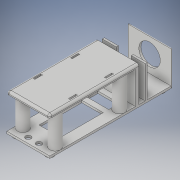
# Autodesk Inventor part: TestingPlatform
Saved by Autodesk Inventor 2017 (Build 210142000, 142)
## iProperties
Created: 2018-05-20
Part Number: TestingPlatform
Material: Generic
Document SubType Name: Modeling
Designer: Arthur
Density: 1 g/cm^3
Appearance: Default
Author: Arthur
Autodesk Inventor part; units mm, degrees
ref_plane "YZ Plane" through (0, 0, 0) normal (1, 0, 0) x (0, 1, 0)
ref_plane "XZ Plane" through (0, 0, 0) normal (0, 1, 0) x (-1, 0, 0)
ref_plane "XY Plane" through (0, 0, 0) normal (0, 0, 1) x (1, 0, 0)
sketch "Sketch1" plane through (0, 0, 0) normal (0, 1, 0) x (-1, 0, 0)
  line L0 (-20, 57.5) -> (20, 57.5)
  line L1 (20, 57.5) -> (20, -57.5)
  line L2 (20, -57.5) -> (-20, -57.5)
  line L3 (-20, -57.5) -> (-20, 57.5)
  line L4 (-20, 57.5) -> (20, -57.5) construction
  line L5 (20, 57.5) -> (-20, -57.5) construction
  point P0 (0, 0)
  dimension "d0" = 40
  dimension "d1" = 115
  constraints: 12 end point, 2 midpoint, 2 parallel, 1 horizontal, 1 perpendicular
  measures "d0" distance of L1.end L2.end
  measures "d1" distance of L0.end L1.end
extrude "Extrusion1" add sketch "Sketch1" along normal blind 2
sketch "Sketch3" plane through (0, 2, 0) normal (0, 1, 0) x (1, 0, 0)
  line L0 (-20, 57.5) -> (-20, -57.5) projected
  line L1 (-20, -57.5) -> (-20, -47.5)
  line L2 (-20, 22.4101) -> (-20, 12.4101)
  line L3 (-20, -47.5) -> (-15, -47.5)
  line L4 (-20, 12.4101) -> (-15, 12.4101)
  line L5 (20, -47.5) -> (15, -47.5)
  circle A0 centre (15, -47.5) radius 5
  circle A1 centre (15, 12.4101) radius 5
  line L6 (20, -57.5) -> (20, 57.5) projected
  circle A2 centre (-15, 12.4101) radius 5
  circle A3 centre (-15, -47.5) radius 5
  line L7 (-20, 22.4101) -> (20, 22.4101)
  line L8 (20, 22.4101) -> (20, 25.4101)
  line L9 (20, 25.4101) -> (-20, 25.4101)
  line L10 (-20, 25.4101) -> (-20, 22.4101)
  line L11 (-20, 25.4101) -> (-20, 31.4101)
  line L12 (-20, 31.4101) -> (-7, 31.4101)
  line L13 (-7, 31.4101) -> (-7, 33.4101)
  line L14 (-7, 33.4101) -> (-20, 33.4101)
  line L15 (-20, 33.4101) -> (-20, 31.4101)
  line L16 (20, 31.4101) -> (7, 31.4101)
  line L17 (7, 31.4101) -> (7, 33.4101)
  line L18 (7, 33.4101) -> (20, 33.4101)
  line L19 (20, 33.4101) -> (20, 31.4101)
  line L20 (20, 57.5) -> (-20, 57.5) projected
  line L21 (20, 57.5) -> (-20, 57.5)
  line L22 (-20, 57.5) -> (-20, 55.5)
  line L23 (-20, 55.5) -> (20, 55.5)
  line L24 (20, 55.5) -> (20, 57.5)
  point P0 (0, 0)
  dimension "d17" = 10
  dimension "d18" = 10
  dimension "d19" = 5
  dimension "d21" = 5
  dimension "d22" = 5
  dimension "d23" = 40
  dimension "d24" = 3
  dimension "d25" = 6
  dimension "d26" = 13
  dimension "d27" = 2
  dimension "d28" = 13
  dimension "d29" = 2
  dimension "d30" = 40
  dimension "d31" = 2
  constraints: 44 end point, 8 parallel, 7 horizontal, 5 point on line, 4 perpendicular, 3 coincident, 3 horizontal alignment, 1 centre point, 1 tangent, 6 other
  measures "d17" distance of L0.end L1.end
  measures "d18" distance of L2.start L2.end
  measures "d19" distance of L1.end L3.end
  measures "d21" distance of L2.end L4.end
  measures "d22" distance of L5.start L5.end
  measures "d23" distance of L9.end L8.end
  measures "d24" distance of L8.end L7.end
  measures "d25" distance of L9.end L11.end
  measures "d26" distance of L14.end L13.end
  measures "d27" distance of L13.end L12.end
  measures "d28" distance of L17.end L18.end
  measures "d29" distance of L16.end L17.end
  measures "d30" distance of L23.end L22.end
  measures "d31" distance of L22.end L21.end
extrude "Extrusion2" add sketch "Sketch3" along normal blind 30 contours L20 L6 L23 L0 | L14 L13 L12 L0 | L6 L16 L17 L18 | L9 L6 L7 L0 | A0 | A1 | A2 | A3
sketch "Sketch5" plane through (-15, 32, -12.4101) normal (0, 1, 0) x (1, 0, 0)
  line L0 (35, 13) -> (-5, 13) projected
  line L1 (35, 45.0899) -> (35, -69.9101) projected
  line L2 (-5, 13) -> (35, 13)
  line L3 (35, 13) -> (35, -69.9101)
  line L4 (35, -69.9101) -> (-5, -69.9101)
  line L5 (-5, -69.9101) -> (-5, 13)
  point P0 (15, -12.4101)
  constraints: 8 end point, 2 parallel, 1 horizontal, 1 perpendicular
extrude "Extrusion3" add sketch "Sketch5" along normal blind 3
sketch "Sketch6" plane through (20, 0, -57.5) normal (0, 0, -1) x (-1, 0, 0)
  line L0 (40, 35) -> (0, 35) projected
  circle A0 centre (20, 17.5) radius 10
  point P0 (20, 0)
  dimension "d37" = 20
  constraints: 1 centre point
  measures "d37" diameter of A0
extrude "Extrusion4" cut sketch "Sketch6" against normal blind 2
sketch "Sketch7" plane through (0, 2, 0) normal (0, 1, 0) x (1, 0, 0)
  line L0 (20, -47.5) -> (20, 12.4101) projected
  circle A0 centre (-15, -47.5) radius 5 projected
  line L1 (10, 2.4101) -> (-10, 2.4101)
  line L2 (-10, 2.4101) -> (-10, -37.5)
  line L3 (-10, -37.5) -> (10, -37.5)
  line L4 (10, -37.5) -> (10, 2.4101)
  point P0 (0, 0)
  point P1 (-20, -47.5)
  constraints: 8 end point, 2 parallel, 1 horizontal, 1 horizontal alignment, 1 perpendicular
extrude "Extrusion5" cut sketch "Sketch7" against normal through all contours L4 L3 L2 L1
fillet "Fillet1" radius 2 1 edges at (-20, 35, 16.045)
fillet "Fillet2" radius 2 1 edges at (20, 35, 16.045)
fillet "Fillet3" radius 2 3 edges at (0, 32, -57.5) (-20, 16, -57.5) (20, 16, -57.5)
fillet "Fillet4" radius 2 5 edges at (0, 35, 57.5) (19.4142, 34.4142, 57.5) (20, 32.5, 57.5) (-19.4142, 34.4142, 57.5) (-20, 32.5, 57.5)
sketch "Sketch8" plane through (0, 2, 0) normal (0, 1, 0) x (1, 0, 0)
  circle A0 centre (-15, -47.5) radius 5 projected
  circle A1 centre (-5, -52.5) radius 2.5
  circle A2 centre (15, -47.5) radius 5 projected
  circle A3 centre (5, -52.5) radius 2.5
  point P0 (0, 0)
  point P1 (-20, -47.5)
  point P2 (20, -47.5)
  dimension "d52" = 5
  dimension "d55" = 5
  constraints: 2 centre point, 2 horizontal alignment
  measures "d52" diameter of A1
  measures "d55" diameter of A3
extrude "Extrusion6" cut sketch "Sketch8" against normal through all contours A1 | A3
sketch "Sketch9" plane through (-15, 35, -12.4101) normal (0, 1, 0) x (1, 0, 0)
  line L0 (-3, -67.9101) -> (-3, 13) projected
  line L1 (-1, -7) -> (-1.5, -7)
  line L2 (-1.5, -7) -> (0, -7)
  line L3 (0, -7) -> (0, -14)
  line L4 (0, -14) -> (-1.5, -14)
  line L5 (-1.5, -14) -> (-1.5, -7)
  line L6 (31, -7) -> (31.5, -7)
  line L7 (31.5, -7) -> (30, -7)
  line L8 (30, -7) -> (30, -14)
  line L9 (30, -14) -> (31.5, -14)
  line L10 (31.5, -14) -> (31.5, -7)
  line L11 (-3, -67.9101) -> (-1.5, -67.9101)
  line L12 (33, -67.9101) -> (-3, -67.9101) projected
  line L13 (-1.5, -47.9101) -> (-2.25, -47.9101)
  line L14 (-2.25, -47.9101) -> (-0.75, -47.9101)
  line L15 (-0.75, -47.9101) -> (-0.75, -40.9101)
  line L16 (-0.75, -40.9101) -> (-2.25, -40.9101)
  line L17 (-2.25, -40.9101) -> (-2.25, -47.9101)
  line L18 (30.75, -47.9101) -> (31.875, -47.9101)
  line L19 (31.875, -47.9101) -> (30.375, -47.9101)
  line L20 (30.375, -47.9101) -> (30.375, -40.9101)
  line L21 (30.375, -40.9101) -> (31.875, -40.9101)
  line L22 (31.875, -40.9101) -> (31.875, -47.9101)
  point P0 (15, -12.4101)
  dimension "d61" = 1.5
  dimension "d62" = 7
  dimension "d65" = 1.5
  dimension "d66" = 7
  dimension "d68" = 1.5
  dimension "d69" = 7
  dimension "d71" = 1.5
  dimension "d72" = 7
  constraints: 42 end point, 8 parallel, 6 horizontal, 4 perpendicular, 1 point on line
  measures "d61" distance of L3.end L4.end
  measures "d62" distance of L2.end L3.end
  measures "d65" distance of L9.end L8.end
  measures "d66" distance of L8.end L7.end
  measures "d68" distance of L16.end L15.end
  measures "d69" distance of L15.end L14.end
  measures "d71" distance of L20.end L21.end
  measures "d72" distance of L19.end L20.end
extrude "Extrusion7" cut sketch "Sketch9" against normal blind 3
sketch "Sketch11" plane through (0, 2, 0) normal (0, 1, 0) x (1, 0, 0)
  line L0 (-10, -37.5) -> (-10, 2.4101) projected
  line L1 (10, 2.4101) -> (10, -37.5) projected
  line L2 (10, 7.4101) -> (-10, 7.4101)
  line L3 (-10, 7.4101) -> (-10, 17.4101)
  line L4 (-10, 17.4101) -> (10, 17.4101)
  line L5 (10, 17.4101) -> (10, 7.4101)
  point P0 (0, 0)
  dimension "d76" = 5
  dimension "d77" = 20
  dimension "d78" = 10
  constraints: 8 end point, 2 parallel, 1 horizontal, 1 perpendicular
  measures "d76" distance of L1.start L2.start
  measures "d77" distance of L3.end L4.end
  measures "d78" distance of L2.end L3.end
extrude "Extrusion8" cut sketch "Sketch11" against normal through all
sketch "Sketch12" plane through (0, 0, 0) normal (0, -1, 0) x (1, 0, 0)
  line L0 (20, -55.5) -> (-20, -55.5) projected
  line L1 (-20, -55.5) -> (-15, -55.5)
  line L2 (20, -55.5) -> (20, 57.5) projected
  line L3 (20, 57.5) -> (-20, 57.5) projected
  circle A0 centre (-15, 47.5) radius 5 projected
  circle A1 centre (15, 47.5) radius 5 projected
  circle A2 centre (-15, -50.5) radius 3.5
  circle A3 centre (15, -50.5) radius 3.5
  circle A4 centre (-15, 52.5) radius 3.5
  circle A5 centre (15, 52.5) radius 3.5
  point P0 (0, 0)
  point P1 (-20, 47.5)
  point P2 (20, 47.5)
  dimension "d88" = 7
  dimension "d89" = 7
  dimension "d90" = 7
  dimension "d91" = 7
  constraints: 4 centre point, 2 end point, 2 horizontal alignment, 1 point on line
  measures "d88" diameter of A2
  measures "d89" diameter of A3
  measures "d90" diameter of A4
  measures "d91" diameter of A5
extrude "Extrusion9" add sketch "Sketch12" along normal blind 2 contours A4 A0 | A0 A4 | A5 A1 | A1 A5 | A2 | A3 picked at (-14.3261, 51.3204) picked at (-15.8785, 53.5139) picked at (15.6739, 51.3204) picked at (14.1215, 53.5139)
body "Solid1"
